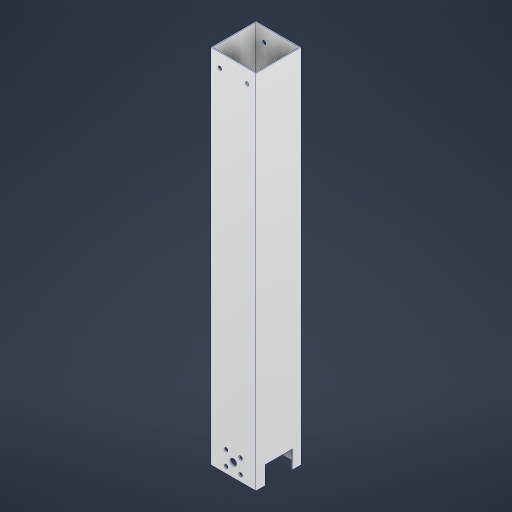
# Autodesk Inventor part: End-Link
Saved by Autodesk Inventor 2023 (Build 270158000, 158)
## iProperties
Created: 2023-08-12
Part Number: End-Link
Material: Aluminum 6061
Document SubType Name: Modeling
Designer: Abhinav
Density: 2.7 g/cm^3
Appearance: Aluminum - Flat
Author: Abhinav
Autodesk Inventor part; units mm, degrees
ref_plane "YZ Plane" through (0, 0, 0) normal (1, 0, 0) x (0, 1, 0)
ref_plane "XZ Plane" through (0, 0, 0) normal (0, 1, 0) x (-1, 0, 0)
ref_plane "XY Plane" through (0, 0, 0) normal (0, 0, 1) x (1, 0, 0)
sketch "Sketch1" plane through (0, 0, 0) normal (0, 1, 0) x (-1, 0, 0)
  line L0 (25, 25) -> (-25, 25)
  line L1 (-25, 25) -> (-25, -25)
  line L2 (-25, -25) -> (25, -25)
  line L3 (25, -25) -> (25, 25)
  line L4 (25, 25) -> (-25, -25) construction
  line L5 (-25, 25) -> (25, -25) construction
  line L6 (24, 24) -> (-24, 24)
  line L7 (-24, 24) -> (-24, -24)
  line L8 (-24, -24) -> (24, -24)
  line L9 (24, -24) -> (24, 24)
  line L10 (24, 24) -> (-24, -24) construction
  line L11 (-24, 24) -> (24, -24) construction
  point P0 (0, 0)
  dimension "d0" = 50
  dimension "d2" = 48
  constraints: 24 end point, 4 midpoint, 4 parallel, 4 perpendicular, 2 horizontal
  measures "d0" distance of L2.end L1.end
  measures "d2" distance of L8.end L7.end
extrude "Extrusion1" add sketch "Sketch1" along normal blind 400
sketch "Sketch3" plane through (25, 0, -25) normal (0, 0, -1) x (-1, 0, 0)
  line L0 (50, 0) -> (50, 400) projected
  line L1 (0, 0) -> (50, 0)
  line L2 (50, 0) -> (50, 30)
  line L3 (50, 30) -> (0, 30)
  line L4 (0, 30) -> (0, 0)
  line L5 (50, 30) -> (0, 0) construction
  line L6 (0, 0) -> (0, 400) projected
  line L7 (50, 0) -> (50, 400) projected
  line L8 (0, 400) -> (50, 400)
  line L9 (50, 400) -> (50, 370)
  line L10 (50, 370) -> (0, 370)
  line L11 (0, 370) -> (0, 400)
  line L12 (0, 400) -> (50, 370) construction
  circle A0 centre (40, 385) radius 2
  line L13 (25, 385) -> (40, 385) construction
  line L14 (25, 385) -> (10, 385) construction
  circle A1 centre (10, 385) radius 2
  circle A2 centre (25, 15) radius 3.5
  line L15 (17, 23) -> (33, 23) construction
  line L16 (33, 23) -> (33, 7) construction
  line L17 (33, 7) -> (17, 7) construction
  line L18 (17, 7) -> (17, 23) construction
  line L19 (17, 23) -> (33, 7) construction
  line L20 (33, 23) -> (17, 7) construction
  circle A3 centre (17, 23) radius 2
  circle A4 centre (33, 23) radius 2
  circle A5 centre (33, 7) radius 2
  circle A6 centre (17, 7) radius 2
  line L21 (25, 15) -> (29.6644, 19.6644) construction
  point P0 (25, 0)
  dimension "d19" = 30
  dimension "d28" = 30
  dimension "d29" = 4
  dimension "d30" = 15
  dimension "d31" = 15
  dimension "d32" = 4
  dimension "d33" = 7
  dimension "d34" = 16
  dimension "d35" = 4
  constraints: 38 end point, 7 centre point, 6 parallel, 5 coincident, 4 horizontal, 4 perpendicular, 3 equal radius, 3 point on line, 2 midpoint
  measures "d19" distance of L2.end L1.end
  measures "d28" distance of L8.end L9.end
  measures "d29" diameter of A0
  measures "d30" distance of L13.start L13.end
  measures "d31" distance of L14.start L14.end
  measures "d32" diameter of A1
  measures "d33" diameter of A2
  measures "d34" distance of L19.end L18.start
  measures "d35" diameter of A3
extrude "Extrusion3" cut sketch "Sketch3" against normal blind 50 contours A0 | A1 | A2 | A3 | A4 | A5 | A6
sketch "Sketch4" plane through (25, 0, 25) normal (1, 0, 0) x (0, 0, -1)
  line L0 (50, 0) -> (0, 0) construction
  line L1 (0, 0) -> (10.1, 0) construction
  line L2 (10.1, 0) -> (40.1, 0)
  line L3 (40.1, 0) -> (40.1, 20)
  line L4 (40.1, 20) -> (10.1, 20)
  line L5 (10.1, 20) -> (10.1, 0)
  point P0 (25, 0)
  dimension "d23" = 10.1
  dimension "d24" = 30
  dimension "d25" = 20
  constraints: 10 end point, 2 parallel, 1 horizontal, 1 perpendicular, 1 point on line
  measures "d23" distance of L0.end L1.end
  measures "d24" distance of L4.end L3.end
  measures "d25" distance of L3.end L2.end
extrude "Extrusion4" cut sketch "Sketch4" against normal blind 10
body "Solid1"
